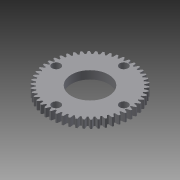
# Autodesk Inventor part: Gear for Extender
Saved by Autodesk Inventor 2013 (Build 170138000, 138)
## iProperties
Created: 2013-01-19
Part Number: Gear for Extender
Material: Generic
Document SubType Name: Modeling
Designer: actoennies
Density: 1 g/cm^3
Mass: 14.8788 g
Surface Area: 83.4995 cm^2
Volume: 14.8788 cm^3
Author: actoennies
Autodesk Inventor part; units mm, degrees
ref_plane "YZ Plane" through (0, 0, 0) normal (1, 0, 0) x (0, 1, 0)
ref_plane "XZ Plane" through (0, 0, 0) normal (0, 1, 0) x (-1, 0, 0)
ref_plane "XY Plane" through (0, 0, 0) normal (0, 0, 1) x (1, 0, 0)
sketch "Sketch1" plane through (0, 0, 0) normal (0, 1, 0) x (-1, 0, 0)
  arc A0 (-15.1548, 1.5123) -> (-15.1548, -1.5123) centre (0, 0) ccw
  arc A1 (-15.1548, -1.5123) -> (-16.0397, -1.8512) centre (-4.8116, -29.8459) ccw
  arc A2 (-16.0397, -1.8512) -> (-18.06, 0.3997) centre (-28.3281, -10.8484) ccw
  arc A3 (-18.06, 0.3997) -> (-19.0035, -0.0313) centre (-4.8116, -29.8459) ccw
  arc A4 (-19.0035, -0.0313) -> (-18.6244, -3.0321) centre (-3.7786, 0.3677) ccw
  arc A5 (-18.6244, -3.0321) -> (-19.4598, -3.4792) centre (-4.8116, -29.8459) ccw
  arc A6 (-19.4598, -3.4792) -> (-21.7463, -1.4992) centre (-30.5236, -13.9456) ccw
  arc A7 (-21.7463, -1.4992) -> (-22.6283, -2.0451) centre (-4.8116, -29.8459) ccw
  arc A8 (-22.6283, -2.0451) -> (-21.8761, -4.9747) centre (-7.5735, 0.2589) ccw
  arc A9 (-21.8761, -4.9747) -> (-22.6489, -5.523) centre (-4.8116, -29.8459) ccw
  arc A10 (-22.6489, -5.523) -> (-25.1655, -3.8452) centre (-32.3137, -17.2935) ccw
  arc A11 (-25.1655, -3.8452) -> (-25.9722, -4.4974) centre (-4.8116, -29.8459) ccw
  arc A12 (-25.9722, -4.4974) -> (-24.8588, -7.3096) centre (-11.3249, -0.3246) ccw
  arc A13 (-24.8588, -7.3096) -> (-25.5567, -7.9504) centre (-4.8116, -29.8459) ccw
  arc A14 (-25.5567, -7.9504) -> (-28.2638, -6.6013) centre (-33.6701, -20.8395) ccw
  arc A15 (-28.2638, -6.6013) -> (-28.9823, -7.3494) centre (-4.8116, -29.8459) ccw
  arc A16 (-28.9823, -7.3494) -> (-27.5252, -9.9999) centre (-14.9735, -1.3737) ccw
  arc A17 (-27.5252, -9.9999) -> (-28.1374, -10.7231) centre (-4.8116, -29.8459) ccw
  arc A18 (-28.1374, -10.7231) -> (-30.9922, -9.7239) centre (-34.5714, -24.5274) ccw
  arc A19 (-30.9922, -9.7239) -> (-31.6113, -10.5562) centre (-4.8116, -29.8459) ccw
  arc A20 (-31.6113, -10.5562) -> (-29.8335, -13.0031) centre (-18.4619, -2.8719) ccw
  arc A21 (-29.8335, -13.0031) -> (-30.3502, -13.7974) centre (-4.8116, -29.8459) ccw
  arc A22 (-30.3502, -13.7974) -> (-33.3077, -13.1639) centre (-35.0033, -28.2992) ccw
  arc A23 (-33.3077, -13.1639) -> (-33.8176, -14.0672) centre (-4.8116, -29.8459) ccw
  arc A24 (-33.8176, -14.0672) -> (-31.7472, -16.272) centre (-21.735, -4.7954) ccw
  arc A25 (-31.7472, -16.272) -> (-32.1602, -17.1248) centre (-4.8116, -29.8459) ccw
  arc A26 (-32.1602, -17.1248) -> (-35.1738, -16.8669) centre (-34.9591, -32.0954) ccw
  arc A27 (-35.1738, -16.8669) -> (-35.5665, -17.827) centre (-4.8116, -29.8459) ccw
  arc A28 (-35.5665, -17.827) -> (-33.236, -19.755) centre (-24.7412, -7.114) ccw
  arc A29 (-33.236, -19.755) -> (-33.539, -20.6528) centre (-4.8116, -29.8459) ccw
  arc A30 (-33.539, -20.6528) -> (-36.5611, -20.7747) centre (-34.4394, -35.8562) ccw
  arc A31 (-36.5611, -20.7747) -> (-36.8304, -21.7764) centre (-4.8116, -29.8459) ccw
  arc A32 (-36.8304, -21.7764) -> (-34.2766, -23.3971) centre (-27.4332, -9.7911) ccw
  arc A33 (-34.2766, -23.3971) -> (-34.4646, -24.3258) centre (-4.8116, -29.8459) ccw
  arc A34 (-34.4646, -24.3258) -> (-37.4477, -24.8255) centre (-33.4525, -39.5221) ccw
  arc A35 (-37.4477, -24.8255) -> (-37.5893, -25.8531) centre (-4.8116, -29.8459) ccw
  arc A36 (-37.5893, -25.8531) -> (-34.8525, -27.1409) centre (-29.7683, -12.7845) ccw
  arc A37 (-34.8525, -27.1409) -> (-34.9227, -28.0858) centre (-4.8116, -29.8459) ccw
  arc A38 (-34.9227, -28.0858) -> (-37.8196, -28.9554) centre (-32.0139, -43.0355) ccw
  arc A39 (-37.8196, -28.9554) -> (-37.8313, -29.9927) centre (-4.8116, -29.8459) ccw
  arc A40 (-37.8313, -29.9927) -> (-34.9547, -30.9273) centre (-31.7099, -16.0469) ccw
  arc A41 (-34.9547, -30.9273) -> (-34.9059, -31.8736) centre (-4.8116, -29.8459) ccw
  arc A42 (-34.9059, -31.8736) -> (-37.6709, -33.0994) centre (-30.1463, -46.3409) ccw
  arc A43 (-37.6709, -33.0994) -> (-37.5525, -34.13) centre (-4.8116, -29.8459) ccw
  arc A44 (-37.5525, -34.13) -> (-34.5815, -34.6967) centre (-33.2273, -19.527) ccw
  arc A45 (-34.5815, -34.6967) -> (-34.4144, -35.6294) centre (-4.8116, -29.8459) ccw
  arc A46 (-34.4144, -35.6294) -> (-37.004, -37.1922) centre (-27.8792, -49.3861) ccw
  arc A47 (-37.004, -37.1922) -> (-36.7574, -38.1997) centre (-4.8116, -29.8459) ccw
  arc A48 (-36.7574, -38.1997) -> (-33.7388, -38.3896) centre (-34.2965, -23.1698) ccw
  arc A49 (-33.7388, -38.3896) -> (-33.4561, -39.294) centre (-4.8116, -29.8459) ccw
  arc A50 (-33.4561, -39.294) -> (-35.8295, -41.169) centre (-25.2483, -52.1231) ccw
  arc A51 (-35.8295, -41.169) -> (-35.4585, -42.1377) centre (-4.8116, -29.8459) ccw
  arc A52 (-35.4585, -42.1377) -> (-32.4398, -41.9478) centre (-34.9007, -26.9179) ccw
  arc A53 (-32.4398, -41.9478) -> (-32.0461, -42.8097) centre (-4.8116, -29.8459) ccw
  arc A54 (-32.0461, -42.8097) -> (-34.1657, -44.9673) centre (-22.295, -54.5089) ccw
  arc A55 (-34.1657, -44.9673) -> (-33.6763, -45.8819) centre (-4.8116, -29.8459) ccw
  arc A56 (-33.6763, -45.8819) -> (-30.7052, -45.3151) centre (-35.0305, -30.7121) ccw
  arc A57 (-30.7052, -45.3151) -> (-30.2065, -46.1208) centre (-4.8116, -29.8459) ccw
  arc A58 (-30.2065, -46.1208) -> (-32.039, -48.5271) centre (-19.0661, -56.5056) ccw
  arc A59 (-32.039, -48.5271) -> (-31.4388, -49.3731) centre (-4.8116, -29.8459) ccw
  arc A60 (-31.4388, -49.3731) -> (-28.5622, -48.4385) centre (-34.6836, -34.4927) ccw
  arc A61 (-28.5622, -48.4385) -> (-27.9665, -49.1753) centre (-4.8116, -29.8459) ccw
  arc A62 (-27.9665, -49.1753) -> (-29.483, -51.7923) centre (-15.6123, -58.082) ccw
  arc A63 (-29.483, -51.7923) -> (-28.7814, -52.5564) centre (-4.8116, -29.8459) ccw
  arc A64 (-28.7814, -52.5564) -> (-26.0447, -51.2686) centre (-33.8657, -38.2001) ccw
  arc A65 (-26.0447, -51.2686) -> (-25.3613, -51.925) centre (-4.8116, -29.8459) ccw
  arc A66 (-25.3613, -51.925) -> (-26.5378, -54.7114) centre (-11.9882, -59.213) ccw
  arc A67 (-26.5378, -54.7114) -> (-25.746, -55.3816) centre (-4.8116, -29.8459) ccw
  arc A68 (-25.746, -55.3816) -> (-23.1923, -53.7609) centre (-32.5895, -41.7756) ccw
  arc A69 (-23.1923, -53.7609) -> (-22.432, -54.3265) centre (-4.8116, -29.8459) ccw
  arc A70 (-22.432, -54.3265) -> (-23.25, -57.2383) centre (-8.251, -59.8809) ccw
  arc A71 (-23.25, -57.2383) -> (-22.3805, -57.804) centre (-4.8116, -29.8459) ccw
  arc A72 (-22.3805, -57.804) -> (-20.05, -55.876) centre (-30.8753, -45.1631) ccw
  arc A73 (-20.05, -55.876) -> (-19.2249, -56.3418) centre (-4.8116, -29.8459) ccw
  arc A74 (-19.2249, -56.3418) -> (-19.6715, -59.3333) centre (-4.4595, -60.0752) ccw
  arc A75 (-19.6715, -59.3333) -> (-18.7379, -59.7855) centre (-4.8116, -29.8459) ccw
  arc A76 (-18.7379, -59.7855) -> (-16.6674, -57.5807) centre (-28.75, -48.3089) ccw
  arc A77 (-16.6674, -57.5807) -> (-15.7904, -57.9394) centre (-4.8116, -29.8459) ccw
  arc A78 (-15.7904, -57.9394) -> (-15.8585, -60.9632) centre (-0.6735, -59.7927) ccw
  arc A79 (-15.8585, -60.9632) -> (-14.8757, -61.2949) centre (-4.8116, -29.8459) ccw
  arc A80 (-14.8757, -61.2949) -> (-13.0978, -58.8479) centre (-26.2472, -51.1636) ccw
  arc A81 (-13.0978, -58.8479) -> (-12.1828, -59.0939) centre (-4.8116, -29.8459) ccw
  arc A82 (-12.1828, -59.0939) -> (-11.8714, -62.1024) centre (3.0472, -59.0379) ccw
  arc A83 (-11.8714, -62.1024) -> (-10.8547, -62.3082) centre (-4.8116, -29.8459) ccw
  arc A84 (-10.8547, -62.3082) -> (-9.3976, -59.6578) centre (-23.4064, -53.6821) ccw
  arc A85 (-9.3976, -59.6578) -> (-8.4589, -59.7871) centre (-4.8116, -29.8459) ccw
  arc A86 (-8.4589, -59.7871) -> (-7.7729, -62.7329) centre (6.6439, -57.8227) ccw
  arc A87 (-7.7729, -62.7329) -> (-6.7385, -62.8097) centre (-4.8116, -29.8459) ccw
  arc A88 (-6.7385, -62.8097) -> (-5.625, -59.9975) centre (-20.2723, -55.8247) ccw
  arc A89 (-5.625, -59.9975) -> (-4.6775, -60.0081) centre (-4.8116, -29.8459) ccw
  arc A90 (-4.6775, -60.0081) -> (-3.6277, -62.8447) centre (10.06, -56.1664) ccw
  arc A91 (-3.6277, -62.8447) -> (-2.5918, -62.7912) centre (-4.8116, -29.8459) ccw
  arc A92 (-2.5918, -62.7912) -> (-1.8396, -59.8617) centre (-16.8944, -57.5576) ccw
  arc A93 (-1.8396, -59.8617) -> (-0.8983, -59.7535) centre (-4.8116, -29.8459) ccw
  arc A94 (-0.8983, -59.7535) -> (0.4988, -62.4361) centre (13.2416, -54.0949) ccw
  arc A95 (0.4988, -62.4361) -> (1.5198, -62.2532) centre (-4.8116, -29.8459) ccw
  arc A96 (1.5198, -62.2532) -> (1.8989, -59.2525) centre (-13.3259, -58.8535) ccw
  arc A97 (1.8989, -59.2525) -> (2.8193, -59.0272) centre (-4.8116, -29.8459) ccw
  arc A98 (2.8193, -59.0272) -> (4.5415, -61.5136) centre (16.1384, -51.6411) ccw
  arc A99 (4.5415, -61.5136) -> (5.5316, -61.2042) centre (-4.8116, -29.8459) ccw
  arc A100 (5.5316, -61.2042) -> (5.5316, -58.1796) centre (-9.6232, -59.6919) ccw
  arc A101 (5.5316, -58.1796) -> (6.4165, -57.8407) centre (-4.8116, -29.8459) ccw
  arc A102 (6.4165, -57.8407) -> (8.4368, -60.0916) centre (18.7049, -48.8435) ccw
  arc A103 (8.4368, -60.0916) -> (9.3803, -59.6605) centre (-4.8116, -29.8459) ccw
  arc A104 (9.3803, -59.6605) -> (9.0012, -56.6598) centre (-5.8445, -60.0596) ccw
  arc A105 (9.0012, -56.6598) -> (9.8366, -56.2127) centre (-4.8116, -29.8459) ccw
  arc A106 (9.8366, -56.2127) -> (12.1231, -58.1927) centre (20.9005, -45.7463) ccw
  arc A107 (12.1231, -58.1927) -> (13.0051, -57.6467) centre (-4.8116, -29.8459) ccw
  arc A108 (13.0051, -57.6467) -> (12.253, -54.7172) centre (-2.0496, -59.9508) ccw
  arc A109 (12.253, -54.7172) -> (13.0258, -54.1689) centre (-4.8116, -29.8459) ccw
  arc A110 (13.0258, -54.1689) -> (15.5424, -55.8467) centre (22.6906, -42.3983) ccw
  arc A111 (15.5424, -55.8467) -> (16.349, -55.1945) centre (-4.8116, -29.8459) ccw
  arc A112 (16.349, -55.1945) -> (15.2356, -52.3823) centre (1.7017, -59.3672) ccw
  arc A113 (15.2356, -52.3823) -> (15.9336, -51.7415) centre (-4.8116, -29.8459) ccw
  arc A114 (15.9336, -51.7415) -> (18.6406, -53.0906) centre (24.0469, -38.8524) ccw
  arc A115 (18.6406, -53.0906) -> (19.3592, -52.3425) centre (-4.8116, -29.8459) ccw
  arc A116 (19.3592, -52.3425) -> (17.9021, -49.692) centre (5.3504, -58.3181) ccw
  arc A117 (17.9021, -49.692) -> (18.5142, -48.9688) centre (-4.8116, -29.8459) ccw
  arc A118 (18.5142, -48.9688) -> (21.369, -49.968) centre (24.9482, -35.1645) ccw
  arc A119 (21.369, -49.968) -> (21.9881, -49.1357) centre (-4.8116, -29.8459) ccw
  arc A120 (21.9881, -49.1357) -> (20.2103, -46.6887) centre (8.8388, -56.82) ccw
  arc A121 (20.2103, -46.6887) -> (20.727, -45.8945) centre (-4.8116, -29.8459) ccw
  arc A122 (20.727, -45.8945) -> (23.6845, -46.528) centre (25.3801, -31.3926) ccw
  arc A123 (23.6845, -46.528) -> (24.1945, -45.6247) centre (-4.8116, -29.8459) ccw
  arc A124 (24.1945, -45.6247) -> (22.124, -43.4199) centre (12.1119, -54.8964) ccw
  arc A125 (22.124, -43.4199) -> (22.5371, -42.5671) centre (-4.8116, -29.8459) ccw
  arc A126 (22.5371, -42.5671) -> (25.5507, -42.825) centre (25.3359, -27.5964) ccw
  arc A127 (25.5507, -42.825) -> (25.9434, -41.8648) centre (-4.8116, -29.8459) ccw
  arc A128 (25.9434, -41.8648) -> (23.6129, -39.9369) centre (15.1181, -52.5778) ccw
  arc A129 (23.6129, -39.9369) -> (23.9158, -39.0391) centre (-4.8116, -29.8459) ccw
  arc A130 (23.9158, -39.0391) -> (26.9379, -38.9172) centre (24.8162, -23.8357) ccw
  arc A131 (26.9379, -38.9172) -> (27.2072, -37.9155) centre (-4.8116, -29.8459) ccw
  arc A132 (27.2072, -37.9155) -> (24.6535, -36.2948) centre (17.81, -49.9007) ccw
  arc A133 (24.6535, -36.2948) -> (24.8415, -35.3661) centre (-4.8116, -29.8459) ccw
  arc A134 (24.8415, -35.3661) -> (27.8245, -34.8664) centre (23.8293, -20.1697) ccw
  arc A135 (27.8245, -34.8664) -> (27.9661, -33.8388) centre (-4.8116, -29.8459) ccw
  arc A136 (27.9661, -33.8388) -> (25.2294, -32.551) centre (20.1451, -46.9074) ccw
  arc A137 (25.2294, -32.551) -> (25.2995, -31.6061) centre (-4.8116, -29.8459) ccw
  arc A138 (25.2995, -31.6061) -> (28.1964, -30.7364) centre (22.3907, -16.6564) ccw
  arc A139 (28.1964, -30.7364) -> (28.2081, -29.6992) centre (-4.8116, -29.8459) ccw
  arc A140 (28.2081, -29.6992) -> (25.3315, -28.7645) centre (22.0867, -43.6449) ccw
  arc A141 (25.3315, -28.7645) -> (25.2827, -27.8183) centre (-4.8116, -29.8459) ccw
  arc A142 (25.2827, -27.8183) -> (28.0477, -26.5924) centre (20.5231, -13.351) ccw
  arc A143 (28.0477, -26.5924) -> (27.9293, -25.5619) centre (-4.8116, -29.8459) ccw
  arc A144 (27.9293, -25.5619) -> (24.9583, -24.9951) centre (23.6041, -40.1649) ccw
  arc A145 (24.9583, -24.9951) -> (24.7912, -24.0624) centre (-4.8116, -29.8459) ccw
  arc A146 (24.7912, -24.0624) -> (27.3809, -22.4997) centre (18.256, -10.3058) ccw
  arc A147 (27.3809, -22.4997) -> (27.1342, -21.4921) centre (-4.8116, -29.8459) ccw
  arc A148 (27.1342, -21.4921) -> (24.1156, -21.3022) centre (24.6733, -36.5221) ccw
  arc A149 (24.1156, -21.3022) -> (23.833, -20.3978) centre (-4.8116, -29.8459) ccw
  arc A150 (23.833, -20.3978) -> (26.2063, -18.5228) centre (15.6251, -7.5687) ccw
  arc A151 (26.2063, -18.5228) -> (25.8353, -17.5541) centre (-4.8116, -29.8459) ccw
  arc A152 (25.8353, -17.5541) -> (22.8167, -17.7441) centre (25.2776, -32.774) ccw
  arc A153 (22.8167, -17.7441) -> (22.4229, -16.8822) centre (-4.8116, -29.8459) ccw
  arc A154 (22.4229, -16.8822) -> (24.5425, -14.7246) centre (12.6719, -5.183) ccw
  arc A155 (24.5425, -14.7246) -> (24.0531, -13.81) centre (-4.8116, -29.8459) ccw
  arc A156 (24.0531, -13.81) -> (21.0821, -14.3767) centre (25.4073, -28.9797) ccw
  arc A157 (21.0821, -14.3767) -> (20.5834, -13.571) centre (-4.8116, -29.8459) ccw
  arc A158 (20.5834, -13.571) -> (22.4159, -11.1648) centre (9.4429, -3.1862) ccw
  arc A159 (22.4159, -11.1648) -> (21.8156, -10.3187) centre (-4.8116, -29.8459) ccw
  arc A160 (21.8156, -10.3187) -> (18.9391, -11.2534) centre (25.0604, -25.1991) ccw
  arc A161 (18.9391, -11.2534) -> (18.3434, -10.5165) centre (-4.8116, -29.8459) ccw
  arc A162 (18.3434, -10.5165) -> (19.8598, -7.8996) centre (5.9892, -1.6099) ccw
  arc A163 (19.8598, -7.8996) -> (19.1583, -7.1354) centre (-4.8116, -29.8459) ccw
  arc A164 (19.1583, -7.1354) -> (16.4215, -8.4233) centre (24.2425, -21.4918) ccw
  arc A165 (16.4215, -8.4233) -> (15.7382, -7.7669) centre (-4.8116, -29.8459) ccw
  arc A166 (15.7382, -7.7669) -> (16.9146, -4.9805) centre (2.3651, -0.4788) ccw
  arc A167 (16.9146, -4.9805) -> (16.1229, -4.3103) centre (-4.8116, -29.8459) ccw
  arc A168 (16.1229, -4.3103) -> (13.5691, -5.931) centre (22.9663, -17.9162) ccw
  arc A169 (13.5691, -5.931) -> (12.8089, -5.3654) centre (-4.8116, -29.8459) ccw
  arc A170 (12.8089, -5.3654) -> (13.6269, -2.4535) centre (-1.3722, 0.1891) ccw
  arc A171 (13.6269, -2.4535) -> (12.7573, -1.8879) centre (-4.8116, -29.8459) ccw
  arc A172 (12.7573, -1.8879) -> (10.4269, -3.8158) centre (21.2521, -14.5288) ccw
  arc A173 (10.4269, -3.8158) -> (9.6017, -3.35) centre (-4.8116, -29.8459) ccw
  arc A174 (9.6017, -3.35) -> (10.0483, -0.3586) centre (-5.1637, 0.3833) ccw
  arc A175 (10.0483, -0.3586) -> (9.1147, 0.0936) centre (-4.8116, -29.8459) ccw
  arc A176 (9.1147, 0.0936) -> (7.0443, -2.1112) centre (19.1269, -11.3829) ccw
  arc A177 (7.0443, -2.1112) -> (6.1672, -1.7525) centre (-4.8116, -29.8459) ccw
  arc A178 (6.1672, -1.7525) -> (6.2354, 1.2714) centre (-8.9496, 0.1008) ccw
  arc A179 (6.2354, 1.2714) -> (5.2525, 1.603) centre (-4.8116, -29.8459) ccw
  arc A180 (5.2525, 1.603) -> (3.4747, -0.844) centre (16.6241, -8.5282) ccw
  arc A181 (3.4747, -0.844) -> (2.5596, -0.598) centre (-4.8116, -29.8459) ccw
  arc A182 (2.5596, -0.598) -> (2.2482, 2.4105) centre (-12.6703, -0.654) ccw
  arc A183 (2.2482, 2.4105) -> (1.2315, 2.6164) centre (-4.8116, -29.8459) ccw
  arc A184 (1.2315, 2.6164) -> (-0.2256, -0.0341) centre (13.7832, -6.0097) ccw
  arc A185 (-0.2256, -0.0341) -> (-1.1642, 0.0952) centre (-4.8116, -29.8459) ccw
  arc A186 (-1.1642, 0.0952) -> (-1.8502, 3.041) centre (-16.2671, -1.8691) ccw
  arc A187 (-1.8502, 3.041) -> (-2.8847, 3.1178) centre (-4.8116, -29.8459) ccw
  arc A188 (-2.8847, 3.1178) -> (-3.9981, 0.3056) centre (10.6491, -3.8671) ccw
  arc A189 (-3.9981, 0.3056) -> (-4.9456, 0.3163) centre (-4.8116, -29.8459) ccw
  arc A190 (-4.9456, 0.3163) -> (-5.9954, 3.1528) centre (-19.6832, -3.5255) ccw
  arc A191 (-5.9954, 3.1528) -> (-7.0314, 3.0994) centre (-4.8116, -29.8459) ccw
  arc A192 (-7.0314, 3.0994) -> (-7.7835, 0.1698) centre (7.2712, -2.1343) ccw
  arc A193 (-7.7835, 0.1698) -> (-8.7249, 0.0616) centre (-4.8116, -29.8459) ccw
  arc A194 (-8.7249, 0.0616) -> (-10.1219, 2.7443) centre (-22.8647, -5.5969) ccw
  arc A195 (-10.1219, 2.7443) -> (-11.143, 2.5614) centre (-4.8116, -29.8459) ccw
  arc A196 (-11.143, 2.5614) -> (-11.5221, -0.4394) centre (3.7027, -0.8384) ccw
  arc A197 (-11.5221, -0.4394) -> (-12.4424, -0.6647) centre (-4.8116, -29.8459) ccw
  arc A198 (-12.4424, -0.6647) -> (-14.1647, 1.8217) centre (-25.7616, -8.0508) ccw
  arc A199 (-14.1647, 1.8217) -> (-15.1548, 1.5123) centre (-4.8116, -29.8459) ccw
  circle A200 centre (-4.8116, -29.8459) radius 26.543 construction
  circle A201 centre (-4.8116, -3.3029) radius 3.302
  circle A202 centre (-4.8116, -56.3889) radius 3.302
  circle A203 centre (21.7314, -29.8459) radius 3.302
  circle A204 centre (-31.3546, -29.8459) radius 3.302
  circle A205 centre (-4.8116, -29.8459) radius 14.605
  dimension "d1" = 53.086
  dimension "d2" = 6.604
  dimension "d3" = 6.604
  dimension "d4" = 6.604
  dimension "d5" = 6.604
  dimension "d6" = 29.21
  constraints: 404 point on circle, 206 centre point, 2 coincident, 601 other
  measures "d1" diameter of A200
  measures "d2" diameter of A201
  measures "d3" diameter of A202
  measures "d4" diameter of A203
  measures "d5" diameter of A204
  measures "d6" diameter of A205
extrude "Extrusion1" add sketch "Sketch1" along normal blind 6.35
body "Solid1"
